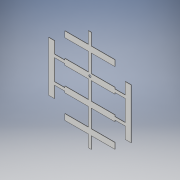
# Autodesk Inventor part: LED Grid v1
Saved by Autodesk Inventor 2019 (Build 230136000, 136)
## iProperties
Created: 2021-08-04
Part Number: LED Grid v1
Material: Generic
Document SubType Name: Modeling
Designer: Lix
Density: 1 g/cm^3
Appearance: Default
Author: Lix
## iProperties of the stored document LED Grid v1_3DPrint.ipt
Created: 2021-08-04
Part Number: LED Grid v1_3DPrint
Material: Generic
Document SubType Name: Modeling
Designer: Lix
Density: 1 g/cm^3
Appearance: Default
Author: Lix
Autodesk Inventor part; units mm, degrees
ref_plane "YZ Plane" through (0, 0, 0) normal (1, 0, 0) x (0, 1, 0)
ref_plane "XZ Plane" through (0, 0, 0) normal (0, 1, 0) x (-1, 0, 0)
ref_plane "XY Plane" through (0, 0, 0) normal (0, 0, 1) x (1, 0, 0)
sketch "Sketch1" plane through (0, 0, 0) normal (0, 0, 1) x (1, 0, 0)
  line L0 (-49.5094, -92.6542) -> (-99.0569, -7.2416)
  line L1 (-99.0569, -7.2416) -> (-49.5094, 79.3458)
  line L2 (-49.5094, 79.3458) -> (49.234, 79.3458)
  line L3 (49.234, 79.3458) -> (97.7547, -6.6542)
  line L4 (97.7547, -6.6542) -> (49.234, -92.6542)
  line L5 (49.234, -92.6542) -> (-49.5094, -92.6542)
  line L6 (-0.1377, 79.3458) -> (-0.1377, -92.6542) construction
  line L7 (-42.6377, 59.0958) -> (42.3623, 59.0958)
  line L8 (42.3623, 59.0958) -> (42.3623, 49.0958)
  line L9 (42.3623, 49.0958) -> (-42.6377, 49.0958)
  line L10 (-42.6377, 49.0958) -> (-42.6377, 59.0958)
  line L11 (-42.6377, 59.0958) -> (42.3623, 49.0958) construction
  line L12 (42.3623, 59.0958) -> (-42.6377, 49.0958) construction
  line L13 (-42.6377, 18.5958) -> (42.3623, 18.5958)
  line L14 (42.3623, 18.5958) -> (42.3623, 8.5958)
  line L15 (42.3623, 8.5958) -> (-42.6377, 8.5958)
  line L16 (-42.6377, 8.5958) -> (-42.6377, 18.5958)
  line L17 (-42.6377, 18.5958) -> (42.3623, 8.5958) construction
  line L18 (42.3623, 18.5958) -> (-42.6377, 8.5958) construction
  line L19 (-42.6377, -21.9042) -> (42.3623, -21.9042)
  line L20 (42.3623, -21.9042) -> (42.3623, -31.9042)
  line L21 (42.3623, -31.9042) -> (-42.6377, -31.9042)
  line L22 (-42.6377, -31.9042) -> (-42.6377, -21.9042)
  line L23 (-42.6377, -21.9042) -> (42.3623, -31.9042) construction
  line L24 (42.3623, -21.9042) -> (-42.6377, -31.9042) construction
  line L25 (-42.6377, -62.4042) -> (42.3623, -62.4042)
  line L26 (42.3623, -62.4042) -> (42.3623, -72.4042)
  line L27 (42.3623, -72.4042) -> (-42.6377, -72.4042)
  line L28 (-42.6377, -72.4042) -> (-42.6377, -62.4042)
  line L29 (-42.6377, -62.4042) -> (42.3623, -72.4042) construction
  line L30 (42.3623, -62.4042) -> (-42.6377, -72.4042) construction
  line L31 (-0.1377, 54.0958) -> (-0.1377, -67.4042) construction
  line L32 (59.8623, 35.8458) -> (69.8623, 35.8458)
  line L33 (69.8623, 35.8458) -> (69.8623, -49.1542)
  line L34 (69.8623, -49.1542) -> (59.8623, -49.1542)
  line L35 (59.8623, -49.1542) -> (59.8623, 35.8458)
  line L36 (59.8623, 35.8458) -> (69.8623, -49.1542) construction
  line L37 (69.8623, 35.8458) -> (59.8623, -49.1542) construction
  line L38 (-60.1377, 35.8458) -> (-70.1377, 35.8458)
  line L39 (-70.1377, 35.8458) -> (-70.1377, -49.1542)
  line L40 (-70.1377, -49.1542) -> (-60.1377, -49.1542)
  line L41 (-60.1377, -49.1542) -> (-60.1377, 35.8458)
  line L42 (-60.1377, 35.8458) -> (-70.1377, -49.1542) construction
  line L43 (-70.1377, 35.8458) -> (-60.1377, -49.1542) construction
  line L44 (-2.6377, 79.3458) -> (2.3623, 79.3458)
  line L45 (2.3623, 79.3458) -> (2.3623, -92.6542)
  line L46 (2.3623, -92.6542) -> (-2.6377, -92.6542)
  line L47 (-2.6377, -92.6542) -> (-2.6377, 79.3458)
  line L48 (-60.1377, 16.0958) -> (59.8623, 16.0958)
  line L49 (59.8623, 16.0958) -> (59.8623, 11.0958)
  line L50 (59.8623, 11.0958) -> (-60.1377, 11.0958)
  line L51 (-60.1377, 11.0958) -> (-60.1377, 16.0958)
  line L52 (-60.1377, -24.4042) -> (59.8623, -24.4042)
  line L53 (59.8623, -24.4042) -> (59.8623, -29.4042)
  line L54 (59.8623, -29.4042) -> (-60.1377, -29.4042)
  line L55 (-60.1377, -29.4042) -> (-60.1377, -24.4042)
  point P0 (-0.1377, 13.5958)
  point P1 (-0.1377, -26.9042)
  point P2 (-0.1377, -6.6542)
  point P3 (64.8623, -6.6542)
  point P4 (64.8623, -6.6542)
  point P5 (-65.1377, -6.6542)
  point P6 (-65.1377, -6.6542)
  point P7 (-0.1377, 79.3458)
  point P8 (-0.1377, 49.0958)
  point P9 (59.8623, 13.5958)
  point P10 (-42.6377, 13.5958)
  point P11 (59.8623, -26.9042)
  point P12 (-0.1377, -26.9042)
  dimension "d0" = 172
  dimension "d12" = 85
  dimension "d13" = 10
  dimension "d16" = 40.5
  dimension "d21" = 20.25
  dimension "d22" = 20.25
  dimension "d23" = 30.5
  dimension "d24" = 10
  dimension "d25" = 85
  dimension "d26" = 120.103
  dimension "d27" = 65
  dimension "d28" = 5
  dimension "d29" = 5
  dimension "d30" = 5
  constraints: 112 end point, 23 midpoint, 10 parallel, 7 collinear, 6 horizontal, 6 symmetric about line, 5 perpendicular, 4 equal length, 3 horizontal alignment, 2 vertical, 1 vertical alignment, 32 other
  measures "d0" distance between parallel lines of L5 L2
  measures "d12" distance of L8.end L9.end
  measures "d13" distance of L7.end L8.end
  measures "d16" distance of L7.start L13.start
  measures "d21" distance between parallel lines of L7 L2
  measures "d22" distance between parallel lines of L5 L27
  measures "d23" distance between parallel lines of L13 L9
  measures "d24" distance of L33.end L34.end
  measures "d25" distance of L32.end L33.end
  measures "d26" angle of L0 L1
  measures "d27" distance of point (64.862, -6.654) point (-0.138, -6.654)
  measures "d28" distance of L44.start L44.end
  measures "d29" distance of L48.end L49.end
  measures "d30" distance of L52.end L53.end
extrude "Extrusion1" add sketch "Sketch1" along normal blind 0.5 contours L47 L27 L45 L5 | L47 L25 L45 L27 | L27 L28 L25 L47 | L2 L45 L7 L47 | L45 L25 L26 L27 | L47 L21 L45 L25 | L47 L9 L10 L7 | L7 L45 L9 L47 | L47 L54 L45 L21 | L21 L22 L54 L47 | L7 L8 L9 L45 | L9 L45 L13 L47 | L45 L54 L20 L21 | L54 L22 L52 L47 | L47 L52 L45 L54 | L47 L48 L16 L13 | L13 L45 L48 L47 | L45 L52 L20 L54 | L54 L41 L52 L22 | L52 L22 L19 L47 | L47 L19 L45 L52 | L13 L14 L48 L45 | L48 L45 L50 L47 | L47 L50 L16 L48 | L20 L52 L35 L54 | L45 L19 L20 L52 | L41 L40 L39 L38 | L47 L15 L45 L19 | L48 L14 L50 L45 | L16 L50 L41 L48 | L50 L45 L15 L47 | L47 L15 L16 L50 | L35 L32 L33 L34 | L48 L35 L50 L14 | L50 L14 L15 L45
sketch "Sketch2" plane through (0, 0, 0.5) normal (0, 0, 1) x (1, 0, 0)
  circle A0 centre (0, 13.9746) radius 2
  point P0 (0, 0)
  dimension "d33" = 4
  constraints: 1 centre point
  measures "d33" diameter of A0
extrude "Extrusion2" cut sketch "Sketch2" against normal blind 10
body "Solid1"
